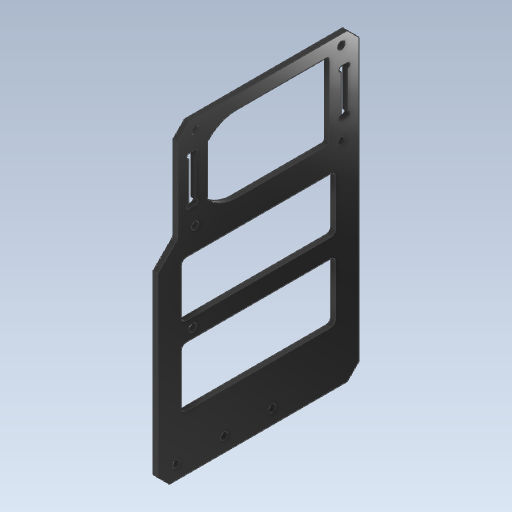
# Autodesk Inventor part: Trunk_upper_side_frame
Saved by Autodesk Inventor 2020 (Build 240168000, 168)
## iProperties
Part Number: Trunk_upper_side_frame
Material: GFRP
Document SubType Name: Modeling
Designer: Masato Kubotera
Density: 1.75 g/cm^3
Appearance: 低 光沢 - 黒
Mass: 19.6924 g
Surface Area: 134.658 cm^2
Volume: 11.2528 cm^3
Description: GFRP T2
Author: Masato Kubotera
Autodesk Inventor part; units mm, degrees
ref_plane "YZ Plane" through (0, 0, 0) normal (1, 0, 0) x (0, 1, 0)
ref_plane "XZ Plane" through (0, 0, 0) normal (0, 1, 0) x (-1, 0, 0)
ref_plane "XY Plane" through (0, 0, 0) normal (0, 0, 1) x (1, 0, 0)
derived "Trunk_basis.ipt"
sketch "スケッチ1" plane through (0, 0, 0) normal (0, 1, 0) x (-1, 0, 0)
  line L0 (0, 22) -> (0, -142.9) construction
  circle A0 centre (5, 0) radius 10.5 construction
  line L1 (-7, 16) -> (36, 16) construction
  line L2 (36, 16) -> (36, -16) construction
  line L3 (36, -16) -> (-7, -16) construction
  line L4 (-7, -16) -> (-7, 16) construction
  line L5 (-7, 16) -> (36, -16) construction
  line L6 (36, 16) -> (-7, -16) construction
  line L7 (33, 13.5) -> (6, 13.5) construction
  line L8 (6, 13.5) -> (6, -13.5) construction
  line L9 (6, -13.5) -> (33, -13.5) construction
  line L10 (33, -13.5) -> (33, 13.5) construction
  line L11 (33, 13.5) -> (6, -13.5) construction
  line L12 (6, 13.5) -> (33, -13.5) construction
  line L13 (-7, 0) -> (36, 0) construction
  arc A1 (5, 16) -> (-7, 10.583) centre (5, 0) ccw construction
  line L14 (43.75, -16.25) -> (5, -16.25) projected
  line L15 (5, 16.25) -> (43.75, 16.25) projected
  line L16 (44.75, 15.25) -> (44.75, -15.25) projected
  arc A2 (5, 16.25) -> (-6.7376, 11.2379) centre (5, 0) ccw projected
  arc A3 (-6.7376, 11.2379) -> (-7.25, 9.9174) centre (-6.2711, 10.2972) ccw projected
  circle A4 centre (6, 13.5) radius 1.35 construction
  line L17 (19.5, 13.5) -> (19.5, -13.5) construction
  circle A5 centre (33, 13.5) radius 1.35 construction
  line L18 (-15, 22) -> (-20, 17) projected
  line L19 (-20, 17) -> (-20, -19) projected
  line L20 (-20, -19) -> (-28.5, -27.5) projected
  line L21 (-28.5, -27.5) -> (-28.5, -103) projected
  line L22 (57.5, -22.5) -> (57.5, 17) projected
  line L23 (57.5, 17) -> (52.5, 22) projected
  line L24 (52.5, 22) -> (-15, 22) projected
  line L25 (-35.5597, -116.5529) -> (-28.5, -142.9) projected
  line L26 (-16, -139) -> (-16, -94) construction
  line L27 (-7.5, -140.4849) -> (-7.5, -142.9) projected
  line L28 (-7.5, -142.9) -> (7.5, -142.9) projected
  line L29 (7.5, -140.4849) -> (7.5, -142.9) projected
  arc A6 (-7.5, -140.4849) -> (-8.9849, -139) centre (-8.2425, -139.7425) ccw projected
  line L30 (-17.5, -138.9955) -> (-17.5, -133) construction
  line L31 (-19, -133) -> (-16, -133) construction
  line L32 (-19, -133) -> (-19, -139) construction
  line L33 (-16, -133) -> (-16, -139) construction
  line L34 (-15, 22) -> (-10, 22) construction
  line L35 (-10, 22) -> (-10, -22) construction
  line L36 (-10, -22) -> (-15, -22) construction
  line L37 (-15, -22) -> (-15, 22) construction
  line L38 (-15, 22) -> (-10, -22) construction
  line L39 (-10, 22) -> (-15, -22) construction
  line L40 (-12.5, 22) -> (-12.5, -22) construction
  line L41 (-10, 0) -> (-15, 0) construction
  circle A7 centre (-12.5, 17.75) radius 1.6 projected
  line L42 (-15, 10) -> (-12.5, 10) construction
  line L43 (-12.5, 10) -> (-12.5, -10) construction
  line L44 (-12.5, -10) -> (-15, -10) construction
  line L45 (-15, -10) -> (-15, 10) construction
  line L46 (-15, 10) -> (-12.5, -10) construction
  line L47 (-12.5, 10) -> (-15, -10) construction
  line L48 (-12.25, 10.25) -> (-15.25, 10.25) projected
  line L49 (-15.25, 8.15) -> (-15.25, -8.15) projected
  line L50 (-15.25, -10.25) -> (-12.25, -10.25) projected
  line L51 (-12.25, -8.15) -> (-12.25, 8.15) projected
  line L52 (-12.25, 10.25) -> (-15.25, -10.25) construction
  line L53 (-15.25, 10.25) -> (-12.25, -10.25) construction
  arc A8 (-15.25, 10.25) -> (-15.25, 8.15) centre (-15.25, 9.2) ccw projected
  line L54 (-13.75, 10) -> (-13.75, -10) construction
  arc A9 (-12.25, 8.15) -> (-12.25, 10.25) centre (-12.25, 9.2) ccw projected
  circle A10 centre (-12.5, -17.75) radius 1.6 projected
  arc A11 (-15.25, -8.15) -> (-15.25, -10.25) centre (-15.25, -9.2) ccw projected
  arc A12 (-12.25, -10.25) -> (-12.25, -8.15) centre (-12.25, -9.2) ccw projected
  line L55 (36, 14.4) -> (44.5, 14.4) construction
  line L56 (44.5, 14.4) -> (44.5, -14.4) construction
  line L57 (36, -14.4) -> (44.5, -14.4) construction
  line L58 (49.95, 7.95) -> (49.95, -7.95) projected
  line L59 (52.5, 0) -> (47.5, 0) construction
  line L60 (47.5, 22) -> (52.5, 22) construction
  line L61 (52.55, -7.95) -> (52.55, 7.95) projected
  line L62 (51.25, 10) -> (51.25, -10) construction
  line L63 (52.5, 10) -> (50, -10) construction
  line L64 (52.5, -10) -> (50, -10) construction
  line L65 (52.5, 10) -> (52.5, -10) construction
  line L66 (50, 10) -> (52.5, -10) construction
  line L67 (49.95, -10.05) -> (52.55, -10.05) projected
  line L68 (49.95, 10.05) -> (52.55, -10.05) construction
  line L69 (52.55, 10.05) -> (49.95, -10.05) construction
  line L70 (52.5, -22) -> (47.5, -22) construction
  line L71 (47.5, 22) -> (52.5, -22) construction
  line L72 (52.5, 22) -> (52.5, -22) construction
  line L73 (52.5, 22) -> (47.5, -22) construction
  line L74 (50, 22) -> (50, -22) construction
  line L75 (47.5, -22) -> (47.5, 22) construction
  circle A13 centre (50, -17.75) radius 1.6 projected
  arc A14 (52.55, -10.05) -> (52.55, -7.95) centre (52.55, -9) ccw projected
  line L76 (50, -10) -> (50, 10) construction
  arc A15 (49.95, -7.95) -> (49.95, -10.05) centre (49.95, -9) ccw projected
  arc A16 (49.95, 10.05) -> (49.95, 7.95) centre (49.95, 9) ccw projected
  arc A17 (52.55, 7.95) -> (52.55, 10.05) centre (52.55, 9) ccw projected
  line L77 (50, 10) -> (52.5, 10) construction
  line L78 (52.55, 10.05) -> (49.95, 10.05) projected
  circle A18 centre (50, 17.75) radius 1.6 projected
  circle A19 centre (5, 0) radius 16 construction
  arc A20 (-6.7376, -11.2379) -> (5, -16.25) centre (5, 0) ccw projected
  arc A21 (-7.25, -9.9174) -> (-6.7376, -11.2379) centre (-6.2711, -10.2972) ccw projected
  line L79 (-7.25, -9.9174) -> (-7.25, 9.9174) projected
  line L80 (17.5, -138.9955) -> (17.5, -133) construction
  line L81 (19, -133) -> (19, -139) construction
  line L82 (16, -133) -> (16, -139) construction
  line L83 (19, -133) -> (16, -133) construction
  circle A22 centre (6, -13.5) radius 1.35 projected
  circle A23 centre (33, -13.5) radius 1.35 projected
  line L84 (-25.5, -142.9) -> (-7.5, -142.9) construction
  line L85 (25.5, -142.9) -> (7.5, -142.9) construction
  line L86 (-23.5, -22.5) -> (57.5, -22.5) construction
  line L87 (57.5, -22.5) -> (57.5, -103) projected
  circle A24 centre (-13.5, -55) radius 1.75 projected
  line L88 (-16.5, -59) -> (45.5, -59) projected
  line L89 (47.5, -61) -> (47.5, -82.5) projected
  line L90 (45.5, -84.5) -> (-16.5, -84.5) projected
  line L91 (-18.5, -82.5) -> (-18.5, -61) projected
  line L92 (-18.5, -59) -> (47.5, -84.5) construction
  line L93 (47.5, -59) -> (-18.5, -84.5) construction
  line L94 (-16.5, -27.5) -> (45.5, -27.5) projected
  line L95 (47.5, -29.5) -> (47.5, -49) projected
  line L96 (45.5, -51) -> (-16.5, -51) projected
  line L97 (-18.5, -49) -> (-18.5, -29.5) projected
  line L98 (-18.5, -27.5) -> (47.5, -51) construction
  line L99 (47.5, -27.5) -> (-18.5, -51) construction
  line L100 (-23.5, -108) -> (-28.5, -103) projected
  circle A25 centre (-20.5415, -102) radius 1.6 projected
  line L101 (-25.7227, -96) -> (25.7227, -96) projected
  line L102 (25.7227, -96) -> (34.9603, -112) projected
  line L103 (35.5597, -116.5529) -> (28.5, -142.9) projected
  line L104 (-25.7227, -96) -> (-34.9603, -112) projected
  line L105 (57.5, -103) -> (52.5, -108) projected
  arc A26 (-16.5, -27.5) -> (-18.5, -29.5) centre (-16.5, -29.5) ccw projected
  arc A27 (-18.5, -49) -> (-16.5, -51) centre (-16.5, -49) ccw projected
  arc A28 (45.5, -51) -> (47.5, -49) centre (45.5, -49) ccw projected
  arc A29 (47.5, -29.5) -> (45.5, -27.5) centre (45.5, -29.5) ccw projected
  arc A30 (-16.5, -59) -> (-18.5, -61) centre (-16.5, -61) ccw projected
  arc A31 (-18.5, -82.5) -> (-16.5, -84.5) centre (-16.5, -82.5) ccw projected
  arc A32 (45.5, -84.5) -> (47.5, -82.5) centre (45.5, -82.5) ccw projected
  arc A33 (47.5, -61) -> (45.5, -59) centre (45.5, -61) ccw projected
  line L106 (-23.5, -108) -> (52.5, -108) projected
  line L107 (-25.5, -139) -> (-25.5, -142.9) projected
  line L108 (-25.5, -142.9) -> (-28.5, -142.9) projected
  line L109 (-17.9813, -99.3843) -> (-16.9961, -101.0907) projected
  line L110 (-16.9961, -102.9093) -> (-17.9813, -104.6157) projected
  line L111 (-19.5563, -105.525) -> (-21.5266, -105.525) projected
  line L112 (-23.1016, -104.6157) -> (-24.0868, -102.9093) projected
  line L113 (-24.0868, -101.0907) -> (-23.1016, -99.3843) projected
  line L114 (-21.5266, -98.475) -> (-19.5563, -98.475) projected
  line L115 (-16, -94) -> (16, -94) construction
  arc A34 (-24.0868, -101.0907) -> (-24.0868, -102.9093) centre (-23.5618, -102) ccw projected
  arc A35 (-23.1016, -104.6157) -> (-21.5266, -105.525) centre (-22.0516, -104.6157) ccw projected
  arc A36 (-19.5563, -105.525) -> (-17.9813, -104.6157) centre (-19.0313, -104.6157) ccw projected
  arc A37 (-16.9961, -102.9093) -> (-16.9961, -101.0907) centre (-17.5211, -102) ccw projected
  arc A38 (-17.9813, -99.3843) -> (-19.5563, -98.475) centre (-19.0313, -99.3843) ccw projected
  arc A39 (-21.5266, -98.475) -> (-23.1016, -99.3843) centre (-22.0516, -99.3843) ccw projected
  line L116 (16, -139) -> (16, -94) construction
  line L117 (16, -94) -> (-16, -94) construction
  line L118 (-25.5, -139) -> (-8.9849, -139) projected
  line L119 (25.5, -142.9) -> (28.5, -142.9) projected
  arc A40 (8.9849, -139) -> (7.5, -140.4849) centre (8.2425, -139.7425) ccw projected
  circle A41 centre (29.7641, -115) radius 1.25 projected
  line L120 (33.4891, -124.2803) -> (21.898, -121.1745) projected
  line L121 (29.7641, -115) -> (25.623, -130.4548) projected
  circle A42 centre (29.7641, -115) radius 6 projected
  circle A43 centre (-20.5415, -102) radius 6 construction
  line L122 (1.9319, -109.4824) -> (7.5588, -130.4824) projected
  line L123 (5.6269, -133) -> (-5.6269, -133) projected
  line L124 (5.3151, -110.5176) -> (10.942, -131.5176) projected
  line L125 (12.8739, -133) -> (17.1947, -133) projected
  line L126 (19.1266, -131.5176) -> (24.7535, -110.5176) projected
  line L127 (22.8217, -108) -> (7.2469, -108) projected
  circle A44 centre (25.623, -130.4548) radius 1.25 projected
  circle A45 centre (25.623, -130.4548) radius 6 construction
  line L128 (-1.9319, -109.4824) -> (-7.5588, -130.4824) projected
  arc A46 (1.9319, -109.4824) -> (-1.9319, -109.4824) centre (0, -110) ccw projected
  arc A47 (-7.5588, -130.4824) -> (-5.6269, -133) centre (-5.6269, -131) ccw projected
  arc A48 (5.6269, -133) -> (7.5588, -130.4824) centre (5.6269, -131) ccw projected
  arc A49 (7.2469, -108) -> (5.3151, -110.5176) centre (7.2469, -110) ccw projected
  arc A50 (24.7535, -110.5176) -> (22.8217, -108) centre (22.8217, -110) ccw projected
  arc A51 (17.1947, -133) -> (19.1266, -131.5176) centre (17.1947, -131) ccw projected
  arc A52 (10.942, -131.5176) -> (12.8739, -133) centre (12.8739, -131) ccw projected
  arc A53 (-5.3151, -110.5176) -> (-7.2469, -108) centre (-7.2469, -110) ccw projected
  line L129 (-22.8217, -108) -> (-7.2469, -108) projected
  line L130 (-5.3151, -110.5176) -> (-10.942, -131.5176) projected
  arc A54 (-22.8217, -108) -> (-24.7535, -110.5176) centre (-22.8217, -110) ccw projected
  line L131 (-19.1266, -131.5176) -> (-24.7535, -110.5176) projected
  arc A55 (-19.1266, -131.5176) -> (-17.1947, -133) centre (-17.1947, -131) ccw projected
  line L132 (-12.8739, -133) -> (-17.1947, -133) projected
  arc A56 (-12.8739, -133) -> (-10.942, -131.5176) centre (-12.8739, -131) ccw projected
  circle A57 centre (-29.7641, -115) radius 1.25 projected
  circle A58 centre (-25.623, -130.4548) radius 1.25 projected
  arc A59 (35.5597, -116.5529) -> (34.9603, -112) centre (29.7641, -115) ccw projected
  arc A60 (-34.9603, -112) -> (-35.5597, -116.5529) centre (-29.7641, -115) ccw projected
  arc A61 (-24.0151, -139) -> (-25.5, -140.4849) centre (-24.7575, -139.7425) ccw projected
  line L133 (25.5, -139) -> (25.5, -142.9) projected
  arc A62 (25.5, -140.4849) -> (24.0151, -139) centre (24.7575, -139.7425) ccw projected
  line L134 (25.5, -139) -> (8.9849, -139) projected
  line L135 (21.5266, -98.475) -> (19.5563, -98.475) projected
  line L136 (16.9961, -102.9093) -> (17.9813, -104.6157) projected
  arc A63 (21.5266, -105.525) -> (23.1016, -104.6157) centre (22.0516, -104.6157) ccw projected
  circle A64 centre (20.5415, -102) radius 1.6 projected
  line L137 (24.0868, -101.0907) -> (23.1016, -99.3843) projected
  arc A65 (24.0868, -102.9093) -> (24.0868, -101.0907) centre (23.5618, -102) ccw projected
  line L138 (23.1016, -104.6157) -> (24.0868, -102.9093) projected
  arc A66 (23.1016, -99.3843) -> (21.5266, -98.475) centre (22.0516, -99.3843) ccw projected
  line L139 (19.5563, -105.525) -> (21.5266, -105.525) projected
  arc A67 (19.5563, -98.475) -> (17.9813, -99.3843) centre (19.0313, -99.3843) ccw projected
  arc A68 (17.9813, -104.6157) -> (19.5563, -105.525) centre (19.0313, -104.6157) ccw projected
  line L140 (17.9813, -99.3843) -> (16.9961, -101.0907) projected
  arc A69 (16.9961, -101.0907) -> (16.9961, -102.9093) centre (17.5211, -102) ccw projected
  line L141 (16, -139) -> (16, -94) construction
  circle A70 centre (20.5415, -102) radius 6 construction
  arc A71 (29.5045, -117.5445) -> (31.2612, -117.0738) centre (30.247, -116.802) ccw construction
  line L142 (31.8379, -116.4971) -> (31.2612, -117.0738) construction
  line L143 (29.5045, -117.5445) -> (28.7167, -117.3334) construction
  arc A72 (27.4307, -116.0474) -> (28.7167, -117.3334) centre (28.4449, -116.3192) ccw construction
  line L144 (27.4307, -116.0474) -> (27.2196, -115.2596) construction
  line L145 (27.6903, -113.5029) -> (28.267, -112.9262) construction
  arc A73 (30.0237, -112.4555) -> (28.267, -112.9262) centre (29.2813, -113.198) ccw construction
  arc A74 (27.6903, -113.5029) -> (27.2196, -115.2596) centre (27.9621, -114.5171) ccw construction
  line L146 (30.0237, -112.4555) -> (30.8116, -112.6666) construction
  arc A75 (31.8379, -116.4971) -> (32.3086, -114.7404) centre (31.5662, -115.4829) ccw construction
  arc A76 (32.0975, -113.9526) -> (30.8116, -112.6666) centre (31.0833, -113.6808) ccw construction
  line L147 (32.0975, -113.9526) -> (32.3086, -114.7404) construction
  line L148 (-20.5415, -102) -> (20.5415, -102) construction
  circle A77 centre (0, -102) radius 1.6 projected
  line L149 (0.4078, -104.525) -> (-0.4078, -104.525) projected
  arc A78 (-0.4078, -99.475) -> (-1.9828, -100.3843) centre (-0.9328, -100.3843) ccw projected
  arc A79 (0.4078, -104.525) -> (1.9828, -103.6157) centre (0.9328, -103.6157) ccw projected
  line L150 (2.3906, -102.9093) -> (1.9828, -103.6157) projected
  line L151 (-0.4078, -99.475) -> (0.4078, -99.475) projected
  arc A80 (1.9828, -100.3843) -> (0.4078, -99.475) centre (0.9328, -100.3843) ccw projected
  line L152 (1.9828, -100.3843) -> (2.3906, -101.0907) projected
  arc A81 (2.3906, -102.9093) -> (2.3906, -101.0907) centre (1.8656, -102) ccw projected
  line L153 (-2.3906, -101.0907) -> (-1.9828, -100.3843) projected
  arc A82 (-2.3906, -101.0907) -> (-2.3906, -102.9093) centre (-1.8656, -102) ccw projected
  line L154 (-1.9828, -103.6157) -> (-2.3906, -102.9093) projected
  arc A83 (-1.9828, -103.6157) -> (-0.4078, -104.525) centre (-0.9328, -103.6157) ccw projected
  circle A84 centre (0, -102) radius 1.25 projected
  arc A85 (44.75, 15.25) -> (43.75, 16.25) centre (43.75, 15.25) ccw projected
  arc A86 (43.75, -16.25) -> (44.75, -15.25) centre (43.75, -15.25) ccw projected
  point P0 (0, 0)
  point P1 (14.5, 0)
  point P2 (19.5, 0)
  point P3 (44.75, 16.25)
  point P4 (-7.25, 10.6771)
  point P5 (19.5, 0)
  point P6 (-12.5, 0)
  point P7 (-13.75, 0)
  point P8 (44.75, 14.4)
  point P9 (44.75, -14.4)
  point P10 (51.25, 0)
  point P11 (50, 0)
  point P12 (44.75, -16.25)
  point P13 (14.5, -71.75)
  point P14 (14.5, -39.25)
  point P15 (15.5276, -102)
  point P16 (15.5276, -139)
  point P17 (-18.5063, -98.475)
  point P18 (-16.4711, -102)
  point P19 (-18.5063, -105.525)
  point P20 (-22.5766, -105.525)
  point P21 (-22.5766, -98.475)
  point P22 (-24.6118, -102)
  point P23 (-22.5766, -105.525)
  point P24 (-18.5063, -105.525)
  point P25 (-16.4711, -102)
  point P26 (-18.5063, -98.475)
  point P27 (-22.5766, -98.475)
  point P28 (27.6936, -122.7274)
  point P29 (0, -102.2726)
  point P30 (0, -133)
  point P31 (-7.5, -139)
  point P32 (-22.5766, -98.475)
  point P33 (18.5063, -98.475)
  point P34 (18.5063, -98.475)
  point P35 (22.5766, -105.525)
  point P36 (22.5766, -105.525)
  point P37 (24.6118, -102)
  point P38 (22.5766, -98.475)
  point P39 (22.5766, -98.475)
  point P40 (22.5766, -98.475)
  point P41 (18.5063, -105.525)
  point P42 (16.4711, -102)
  point P43 (16.4711, -102)
  point P44 (18.5063, -105.525)
  point P45 (29.7641, -115)
  point P46 (29.7641, -115)
  point P47 (30.5187, -117.8163)
  point P48 (30.5187, -117.8163)
  point P49 (27.7025, -117.0617)
  point P50 (27.7025, -117.0617)
  point P51 (31.8258, -112.9383)
  point P52 (26.9479, -114.2454)
  point P53 (29.0095, -112.1837)
  point P54 (29.0095, -112.1837)
  point P55 (31.8258, -112.9383)
  point P56 (29.0095, -112.1837)
  point P57 (32.5804, -115.7546)
  point P58 (-1.4578, -99.475)
  point P59 (-1.4578, -99.475)
  point P60 (-1.4578, -99.475)
  point P61 (1.4578, -104.525)
  point P62 (1.4578, -99.475)
  point P63 (1.4578, -99.475)
  point P64 (2.9156, -102)
  point P65 (-2.9156, -102)
  point P66 (-1.4578, -104.525)
  point P67 (-1.4578, -104.525)
  constraints: 6 other
extrude "押し出し1" add sketch "スケッチ1" along normal blind 2 contours L24 L23 L22 L87 L105 L106 L102 L101 L104 L21 L20 L19 L18 | L104 L101 L102 L106 L100 L21 | L109 A37 L110 A36 L111 A35 L112 A34 L113 A39 L114 A38 | A66 L137 A65 L138 A63 L139 A68 L136 A69 L140 A67 L135 | L149 A83 L154 A82 L153 A78 L151 A80 L152 A81 L150 A79
fillet "フィレット1" radius 2 1 edges at (20, 1, -19)
